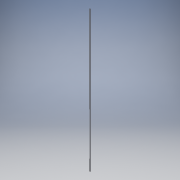
# Autodesk Inventor part: Soporte Horizontal
Saved by Autodesk Inventor 2016 (Build 200138000, 138)
## iProperties
Created: 2015-11-10
Part Number: Soporte Horizontal
Material: Generic
Document SubType Name: Sheet Metal
Designer: serge
Density: 1 g/cm^3
Sheet Metal Rule: Default
Appearance: Valor por defecto
Author: serge
Autodesk Inventor part; units mm, degrees
ref_plane "YZ Plane" through (0, 0, 0) normal (1, 0, 0) x (0, 1, 0)
ref_plane "XZ Plane" through (0, 0, 0) normal (0, 1, 0) x (-1, 0, 0)
ref_plane "XY Plane" through (0, 0, 0) normal (0, 0, 1) x (1, 0, 0)
sketch "Sketch1" plane through (0, 0, 0) normal (0, 0, 1) x (1, 0, 0)
  line L0 (-32.354, 0) -> (11.646, 0)
  line L1 (11.646, 0) -> (11.646, 20)
  line L2 (-32.354, 0) -> (-32.354, 20)
  point P0 (0, 0)
  dimension "d0" = 20
  dimension "d1" = 20
  dimension "d2" = 44
  measures "d0" distance of L0.end L1.end
  measures "d1" distance of L0.start L2.end
  measures "d2" distance of L0.start L0.end
contour flange "Contour Flange1" sketch "Sketch1" thickness 3 bend radius 3 width 933.45 along (0, 0, 1) mid plane no both sides no wall seen from (-32.354, 10, 0) lies toward (-1, 0, 0) curves L2 L0 L1
bend "Bend1"
corner "Corner1"
fillet "Corner Round1" radius 6 4 edges at (-33.854, 20, 933.45) (13.146, 20, 933.45) (-33.854, 20, 0) (13.146, 20, 0)
sketch "Sketch2" plane through (-29.354, -3, 933.45) normal (0, -1, 0) x (1, 0, 0)
  line L0 (0, -933.45) -> (38, -933.45) projected
  line L1 (19, -933.45) -> (19, -858.774)
  arc A0 (14.2375, -858.774) -> (23.7625, -858.774) centre (19, -858.774) ccw
  line L2 (19, -858.774) -> (19, -625.4115)
  arc A1 (23.7625, -625.4115) -> (14.2375, -625.4115) centre (19, -625.4115) ccw
  line L3 (23.7625, -858.774) -> (23.7625, -625.4115)
  line L4 (14.2375, -858.774) -> (14.2375, -625.4115)
  point P0 (29.354, -933.45)
  dimension "distanciaborde" = 74.676
  dimension "d16" = 9.525
  dimension "longguia" = 233.3625
  dimension "d18" = 9.525
  dimension "d19" = 9.525
  dimension "longguia1" = 233.3625
  constraints: 8 end point, 4 point on circle, 2 centre point, 2 coincident, 2 tangent, 1 collinear, 1 midpoint, 1 perpendicular
  measures "distanciaborde" distance of L1.start L1.end
  measures "d16" diameter of A0
  measures "longguia" distance of L2.start L2.end
  measures "d18" diameter of A1
  measures "d19" distance between parallel lines of L3 L4
  measures "longguia1" distance of L3.start L3.end
extrude "Extrusion1" cut sketch "Sketch2" against normal blind 10
pattern_linear "Rectangular Pattern1" count 2 spacing 448.6275 along (0, 0, 1) of "Extrusion1"
equation "\"distanciaborde\" = d_bor2"
equation "\"longguia\" = lon_gui2"
equation "\"longguia1\" = lon_gui2"
equation "\"d25\" = esp_gui2"
equation "\"d3\" = BendReliefWidth"
equation "\"d4\" = BendReliefDepth"
equation "\"d5\" = MinimumRemnant"
equation "\"d6\" = BendRadius"
equation "\"d8\" = BendRadius"
equation "\"d10\" = CornerReliefSize"
equation "\"d11\" = GapSize"
equation "\"d12\" = JacobiRadiusSize"
equation "\"Longitud\" = lon_ho2"
equation "\"BendRadius\" = Thickness"
equation "\"BendReliefWidth\" = Thickness"
equation "\"BendReliefDepth\" = 0.5 * Thickness"
equation "\"CornerReliefSize\" = 4 * Thickness"
equation "\"MinimumRemnant\" = 2 * Thickness"
equation "\"TransitionRadius\" = BendRadius"
equation "\"JacobiRadiusSize\" = Thickness"
equation "\"GapSize\" = Thickness"
equation "\"lon_ho2\" = 933.45"
equation "\"d_bor2\" = 74.676"
equation "\"lon_gui2\" = 233.3625"
equation "\"esp_gui2\" = 448.6275"
equation "\"PE_N\" = 101.6"
equation "\"PE_S\" = 101.6"
equation "\"PE_EO\" = 101.6"
equation "\"T_E\" = 101.6"
equation "\"lon_ve\" = 512.5"
equation "\"n_a\" = 3"
equation "\"t_a\" = 19.05"
equation "\"d_a\" = 128.125"
equation "\"lon_ho\" = 749"
equation "\"d_bor\" = 59.92"
equation "\"lon_gui\" = 187.25"
equation "\"esp_gui\" = 461.25"
equation "\"lon_ve2\" = 498.475"
equation "\"n_a2\" = 3"
equation "\"t_a2\" = 124.61875"
equation "\"d_a2\" = 124.61875"
equation "\"UE_L\" = 2671"
equation "\"UE_A\" = 1025"
equation "\"UE_AN\" = 749"
equation "\"UC_L\" = 1314.45"
equation "\"UC_A\" = 996.95"
equation "\"UC_AN\" = 933.45"
equation "\"A_ET\" = 35"
equation "\"SEP_NS\" = 0"
equation "\"DSEG\" = 0"
equation "\"AEGEP_NS\" = 0"
equation "\"DNS\" = 749"
equation "\"Thickness\" = 3"
body "Solid1"
